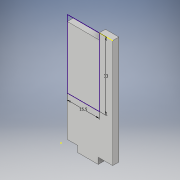
# Autodesk Inventor part: hollow_mount
Saved by Autodesk Inventor 2017.2 (Build 212233000, 233)
## iProperties
Created: 2017-06-15
Part Number: hollow_mount
Material: Generic
Document SubType Name: Modeling
Designer: SandeepSH
Density: 1 g/cm^3
Appearance: Default
Author: SandeepSH
Autodesk Inventor part; units mm, degrees
ref_plane "YZ Plane" through (0, 0, 0) normal (1, 0, 0) x (0, 1, 0)
ref_plane "XZ Plane" through (0, 0, 0) normal (0, 1, 0) x (-1, 0, 0)
ref_plane "XY Plane" through (0, 0, 0) normal (0, 0, 1) x (1, 0, 0)
sketch "Sketch1" plane through (0, 0, 0) normal (0, 0, 1) x (1, 0, 0)
  line L0 (0, 0) -> (25, 0)
  line L1 (25, 0) -> (25, 55.5)
  line L2 (25, 55.5) -> (0, 55.5)
  line L3 (0, 55.5) -> (0, 0)
  dimension "d0" = 25
  dimension "d1" = 55.5
  constraints: 8 end point, 2 parallel, 1 horizontal, 1 perpendicular
  measures "d0" distance of L2.end L1.end
  measures "d1" distance of L1.end L0.end
extrude "Extrusion1" add sketch "Sketch1" along normal blind 3
sketch "Sketch2" plane through (0, 0, 3) normal (0, 0, 1) x (1, 0, 0)
  line L0 (0, 55.5) -> (0, 0) projected
  line L1 (25, 55.5) -> (0, 55.5) projected
  line L2 (0, 0) -> (3, 0)
  line L3 (3, 0) -> (3, 55.5)
  line L4 (3, 55.5) -> (0, 55.5)
  line L5 (0, 55.5) -> (0, 0)
  dimension "d4" = 3
  constraints: 8 end point, 2 parallel, 1 horizontal, 1 perpendicular, 1 point on line
  measures "d4" distance of L4.end L3.end
extrude "Extrusion2" cut sketch "Sketch2" against normal through all
sketch "Sketch3" plane through (0, 0, 3) normal (0, 0, 1) x (1, 0, 0)
  point P0 (0, 0)
sketch "Sketch4" plane through (0, 0, 3) normal (0, 0, 1) x (1, 0, 0)
  line L0 (25, 55.5) -> (3, 55.5) projected
  line L1 (3, 55.5) -> (18.5, 55.5)
  line L2 (18.5, 55.5) -> (18.5, 22.5)
  line L3 (18.5, 22.5) -> (3, 22.5)
  line L4 (3, 22.5) -> (3, 55.5)
  point P0 (0, 0)
  dimension "d7" = 15.5
  dimension "d8" = 33
  constraints: 8 end point, 2 parallel, 1 horizontal, 1 perpendicular
  measures "d7" distance of L2.end L3.end
  measures "d8" distance of L1.end L2.end
sketch "Sketch5" plane through (0, 0, 3) normal (0, 0, 1) x (1, 0, 0)
  line L0 (3, 0) -> (25, 0) projected
  line L1 (8, 0) -> (18, 0)
  line L2 (18, 0) -> (18, 3)
  line L3 (18, 3) -> (8, 3)
  line L4 (8, 3) -> (8, 0)
  line L5 (3, 55.5) -> (3, 0) projected
  line L6 (3, 0) -> (8, 0)
  line L7 (8, 0) -> (8, 3)
  line L8 (8, 3) -> (3, 3)
  line L9 (3, 3) -> (3, 0)
  line L10 (18, 0) -> (25, 0)
  line L11 (25, 0) -> (25, 3)
  line L12 (25, 3) -> (18, 3)
  line L13 (18, 3) -> (18, 0)
  point P0 (0, 0)
  point P1 (3, 22.5)
  dimension "d11" = 10
  dimension "d12" = 3
  dimension "d13" = 5
  constraints: 24 end point, 6 parallel, 3 horizontal, 3 perpendicular, 2 point on line
  measures "d11" distance of L3.end L2.end
  measures "d12" distance of L2.end L1.end
  measures "d13" distance between parallel lines of L5 L4
extrude "Extrusion4" cut sketch "Sketch5" against normal through all contours L5 L8 L4 L0 | L2 L12 L11 L0
sketch "Sketch6" plane through (0, 0, 3) normal (0, 0, 1) x (1, 0, 0)
  line L0 (25, 55.5) -> (3, 55.5) projected
  line L1 (3, 55.5) -> (18.5, 55.5)
  line L2 (18.5, 55.5) -> (18.5, 52.5)
  line L3 (18.5, 52.5) -> (3, 52.5)
  line L4 (3, 52.5) -> (3, 55.5)
  line L5 (18.5, 55.5) -> (18.5, 22.5) projected
  point P0 (0, 0)
  dimension "d16" = 3
  constraints: 8 end point, 2 parallel, 1 collinear, 1 horizontal, 1 perpendicular
  measures "d16" distance of L1.end L2.end
extrude "Extrusion5" cut sketch "Sketch6" against normal through all
body "Solid1"
